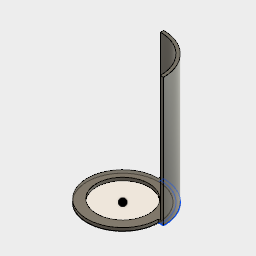
Gelatin_Mold_Remover v2 (Autodesk Fusion 360 design; units mm, degrees)
Autodesk Fusion 360 part; units mm, degrees
sketch "Sketch1" plane through (0, 0, 0) normal (0, 1, 0) x (1, 0, 0)
  circle A0 centre (0, 0) radius 34
  line L0 (0.0039, 39) -> (0.0039, 34)
  line L1 (39, 0.0006) -> (34, 0.0006)
  arc A1 (39, 0.0006) -> (0.0039, 39) centre (0, 0) ccw
  arc A2 (36, 0.0006) -> (0.0039, 36) centre (0, 0) ccw
  dimension "d1" = 68
  measures "d1" diameter of A0
extrude "Extrude1" add sketch "Sketch1" along normal blind 3 contours A0
extrude "Extrude2" add sketch "Sketch1" along normal blind 3 contours A0 L0 L1 A2
extrude "Extrude3" add sketch "Sketch1" along normal blind 123 contours L0 L1 A1 A2
sketch "Sketch2" plane through (0, 3, 0) normal (0, 1, 0) x (-1, 0, 0)
  arc A0 (-0.0039, -34) -> (-34, -0.0006) centre (0, 0) ccw
  line L0 (-34, -0.0006) -> (-36, -0.0006)
  arc A1 (-36, -0.0006) -> (-0.0039, -36) centre (0, 0) ccw
  line L1 (-0.0039, -36) -> (-0.0039, -34)
  circle A2 centre (0, 0) radius 34
  circle A3 centre (0, 0) radius 34
  circle A4 centre (0, 0) radius 25
  dimension "d10" = 9
extrude "Extrude4" cut sketch "Sketch2" against normal blind 3 contours A4
